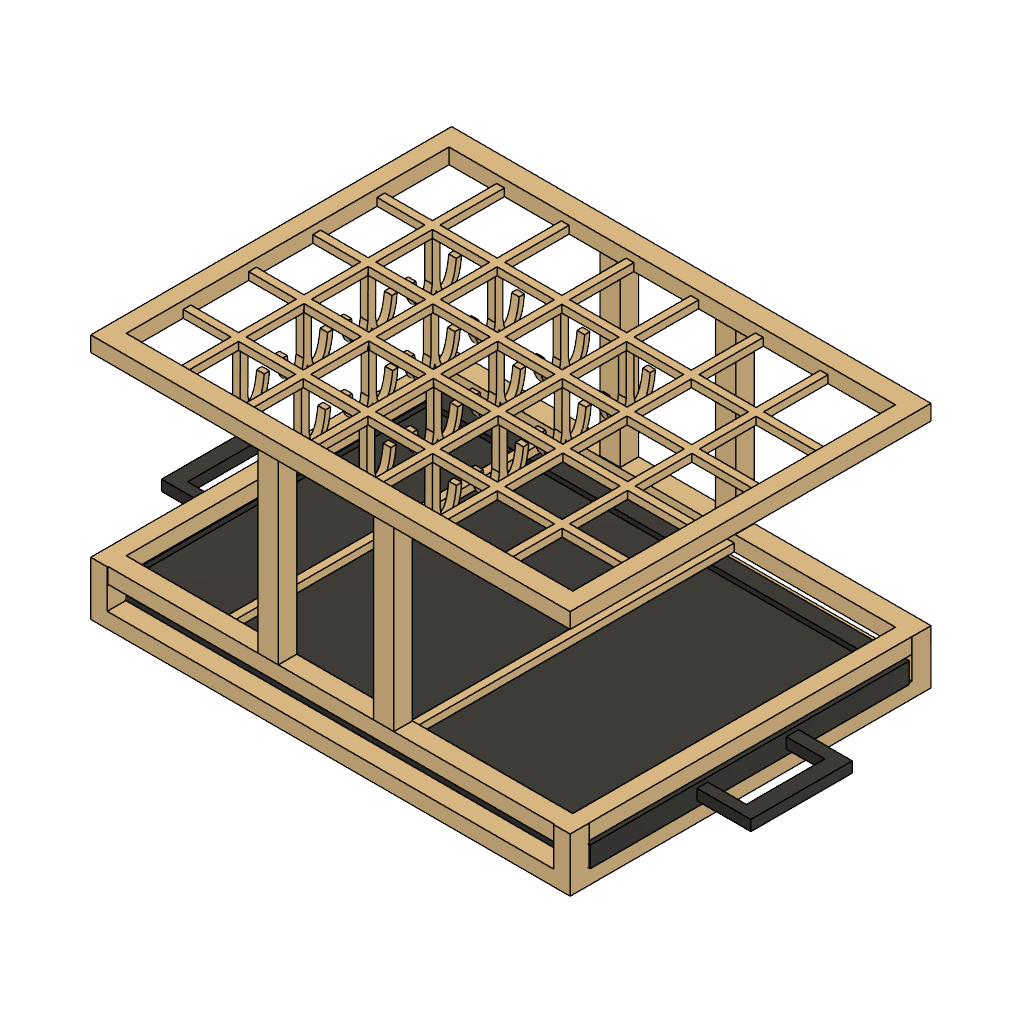
umbrella stand (Autodesk Fusion 360 design; units mm, degrees)
part number: 2026-07-15-13-42-07-009
Autodesk Fusion 360 part; units mm, degrees
note: some values were not read from the file. Chosen so that the rebuilt part matches the saved one: which bodies a step acts on; which face or edge a step refers to.
sketch "Sketch1" plane through (0, 0, 0) normal (0, 1, 0) x (1, 0, 0)
  line L0 (311.1189, -234.2212) -> (-311.1189, -234.2212)
  line L1 (-311.1189, -234.2212) -> (-311.1189, 234.2212)
  line L2 (-311.1189, 234.2212) -> (311.1189, 234.2212)
  line L3 (311.1189, 234.2212) -> (311.1189, -234.2212)
  line L4 (311.1189, -234.2212) -> (-311.1189, 234.2212) construction
  line L5 (-311.1189, -234.2212) -> (311.1189, 234.2212) construction
  line L6 (289.6996, -209.3887) -> (-289.6996, -209.3887)
  line L7 (-289.6996, -209.3887) -> (-289.6996, 209.3887)
  line L8 (-289.6996, 209.3887) -> (289.6996, 209.3887)
  line L9 (289.6996, 209.3887) -> (289.6996, -209.3887)
  line L10 (289.6996, -209.3887) -> (-289.6996, 209.3887) construction
  line L11 (-289.6996, -209.3887) -> (289.6996, 209.3887) construction
  line L12 (289.6996, -209.3887) -> (289.6996, -234.2212)
  line L13 (289.6996, -209.3887) -> (311.1189, -209.3887)
  line L14 (-289.6996, -209.3887) -> (-311.1189, -209.3887)
  line L15 (-311.1189, -209.3887) -> (-311.1189, -234.2212)
  line L16 (-311.1189, -234.2212) -> (-289.6996, -234.2212)
  line L17 (-289.6996, -234.2212) -> (-289.6996, -209.3887)
  line L18 (-289.6996, 209.3887) -> (-311.1189, 209.3887)
  line L19 (-311.1189, 209.3887) -> (-311.1189, 234.2212)
  line L20 (-311.1189, 234.2212) -> (-289.6996, 234.2212)
  line L21 (-289.6996, 234.2212) -> (-289.6996, 209.3887)
  line L22 (289.6996, 209.3887) -> (311.1189, 209.3887)
  line L23 (311.1189, 209.3887) -> (311.1189, 234.2212)
  line L24 (311.1189, 234.2212) -> (289.6996, 234.2212)
  line L25 (289.6996, 234.2212) -> (289.6996, 209.3887)
  constraint horizontal L0
  constraint perpendicular L0 L1
  constraint parallel L0 L2
  constraint parallel L1 L3
  constraint coincident L4 origin
  constraint coincident L5 origin
  constraint horizontal L6
  constraint perpendicular L6 L7
  constraint parallel L6 L8
  constraint parallel L7 L9
  constraint coincident L10 origin
  constraint coincident L11 origin
  constraint coincident L0 L12.end
  constraint perpendicular L0 L12
  constraint coincident L3 L13.end
  constraint perpendicular L3 L13
  constraint horizontal L14
  constraint vertical L15
  constraint horizontal L16
  constraint vertical L17
  constraint horizontal L18
  constraint vertical L19
  constraint horizontal L20
  constraint vertical L21
  constraint horizontal L22
  constraint vertical L23
  constraint horizontal L24
  constraint vertical L25
sketch "Sketch2" plane through (0, 0, 0) normal (0, 1, 0) x (1, 0, 0)
  line L0 (289.429, 6.0189) -> (-289.8763, 6.0189)
  line L1 (-289.8763, 6.0189) -> (-289.8763, 16.0189)
  line L2 (-289.8763, 16.0189) -> (289.429, 16.0189)
  line L3 (289.429, 16.0189) -> (289.429, 6.0189)
  line L4 (78, 210) -> (88, 210)
  line L5 (88, 210) -> (88, -209.6346)
  line L6 (88, -209.6346) -> (78, -209.6346)
  line L7 (78, -209.6346) -> (78, 210)
  line L8 (191.4008, 210) -> (201.4008, 210)
  line L9 (201.4008, 210) -> (201.4008, -209.2657)
  line L10 (201.4008, -209.2657) -> (191.4008, -209.2657)
  line L11 (191.4008, -209.2657) -> (191.4008, 210)
  line L12 (-289.8763, 126.0189) -> (289.429, 126.0189)
  line L13 (289.429, 126.0189) -> (289.429, 116.0189)
  line L14 (289.429, 116.0189) -> (-289.8763, 116.0189)
  line L15 (-289.8763, 116.0189) -> (-289.8763, 126.0189)
  line L16 (289.429, -118.9811) -> (-289.8763, -118.9811)
  line L17 (-289.8763, -118.9811) -> (-289.8763, -108.9811)
  line L18 (-289.8763, -108.9811) -> (289.429, -108.9811)
  line L19 (289.429, -108.9811) -> (289.429, -118.9811)
  line L20 (-42, 210) -> (-42, -209.6346)
  line L21 (-42, -209.6346) -> (-52, -209.6346)
  line L22 (-52, -209.6346) -> (-52, 210)
  line L23 (-52, 210) -> (-42, 210)
  line L24 (-157, 210) -> (-157, -209.6346)
  line L25 (-157, -209.6346) -> (-167, -209.6346)
  line L26 (-167, -209.6346) -> (-167, 210)
  line L27 (-167, 210) -> (-157, 210)
  line L28 (-280, 210) -> (-280, -209.6346)
  line L29 (-280, -209.6346) -> (-290, -209.6346)
  line L30 (-290, -209.6346) -> (-290, 210)
  line L31 (-290, 210) -> (-280, 210)
  line L32 (289.429, 116.0189, 300) -> (-289.8763, 116.0189, 300)
  line L33 (-289.8763, 116.0189, 300) -> (-289.8763, 126.0189, 300)
  line L34 (-289.8763, 126.0189, 300) -> (289.429, 126.0189, 300)
  line L35 (289.429, 126.0189, 300) -> (289.429, 116.0189, 300)
  dimension "d1" = 10
  dimension "d2" = 10
  dimension "d3" = 10
  dimension "d17" = 10
  dimension "d18" = 10
  dimension "d19" = 10
  dimension "d20" = 10
  dimension "d21" = 10
  dimension "d30" = 10
  constraint horizontal L0
  constraint vertical L1
  constraint horizontal L2
  constraint vertical L3
  constraint horizontal L4
  constraint vertical L5
  constraint horizontal L6
  constraint vertical L7
  constraint horizontal L8
  constraint vertical L9
  constraint horizontal L10
  constraint vertical L11
  constraint horizontal L14
  constraint vertical L15
  constraint horizontal L12
  constraint vertical L13
  constraint horizontal L16
  constraint vertical L17
  constraint horizontal L18
  constraint vertical L19
  constraint horizontal L23
  constraint vertical L20
  constraint horizontal L21
  constraint vertical L22
  constraint horizontal L27
  constraint vertical L24
  constraint horizontal L25
  constraint vertical L26
  constraint horizontal L31
  constraint vertical L28
  constraint horizontal L29
  constraint vertical L30
  measures "d1" distance of L0.start L2.end
  measures "d2" distance of L4.start L4.end
  measures "d3" distance of L8.start L8.end
  measures "d17" distance of L13.end L12.end
  measures "d18" distance of L16.start L18.end
  measures "d19" distance of L20.start L22.end
  measures "d20" distance of L24.start L26.end
  measures "d21" distance of L28.start L30.end
  measures "d30" distance of L12.end L13.end
ref_plane "WorkPlane1" through (0, 50, 0) normal (0, 1, 0) x (1, 0, 0)
sketch "Sketch3" plane through (0, 50, 0) normal (0, 1, 0) x (1, 0, 0)
  line L0 (-311.2382, 234.3503) -> (310.9801, 234.3503)
  line L1 (310.9801, 234.3503) -> (310.9801, -233.4061)
  line L2 (310.9801, -233.4061) -> (-311.2382, -233.4061)
  line L3 (-311.2382, -233.4061) -> (-311.2382, 234.3503)
  line L4 (-289.7, 209.4) -> (289.7, 209.4)
  line L5 (289.7, 209.4) -> (289.7, -209.39)
  line L6 (289.7, -209.39) -> (-289.7, -209.39)
  line L7 (-289.7, -209.39) -> (-289.7, 209.4)
  line L8 (310.9801, -233.4061) -> (289.7, -233.4061)
  line L9 (289.7, -233.4061) -> (289.7, -209.39)
  line L10 (289.7, -209.39) -> (310.9801, -209.39)
  line L11 (310.9801, -209.39) -> (310.9801, -233.4061)
  line L12 (-289.7, -209.39) -> (-311.2382, -209.39)
  line L13 (-311.2382, -209.39) -> (-311.2382, -233.4061)
  line L14 (-311.2382, -233.4061) -> (-289.7, -233.4061)
  line L15 (-289.7, -233.4061) -> (-289.7, -209.39)
  line L16 (-289.7, 209.4) -> (-311.2382, 209.4)
  line L17 (-311.2382, 209.4) -> (-311.2382, 234.3503)
  line L18 (-311.2382, 234.3503) -> (-289.7, 234.3503)
  line L19 (-289.7, 234.3503) -> (-289.7, 209.4)
  line L20 (289.7, 209.4) -> (310.9801, 209.4)
  line L21 (310.9801, 209.4) -> (310.9801, 234.3503)
  line L22 (310.9801, 234.3503) -> (289.7, 234.3503)
  line L23 (289.7, 234.3503) -> (289.7, 209.4)
  constraint horizontal L0
  constraint vertical L1
  constraint horizontal L2
  constraint vertical L3
  constraint horizontal L4
  constraint vertical L5
  constraint horizontal L6
  constraint vertical L7
  constraint horizontal L8
  constraint vertical L9
  constraint horizontal L10
  constraint vertical L11
  constraint horizontal L12
  constraint vertical L13
  constraint horizontal L14
  constraint vertical L15
  constraint horizontal L16
  constraint vertical L17
  constraint horizontal L18
  constraint vertical L19
  constraint horizontal L20
  constraint vertical L21
  constraint horizontal L22
  constraint vertical L23
sketch "Sketch4" plane through (0, 50, 0) normal (0, 1, 0) x (1, 0, 0)
  line L0 (-167, 210) -> (-157, 210)
  line L1 (-157, 210) -> (-157, -210)
  line L2 (-157, -210) -> (-167, -210)
  line L3 (-167, -210) -> (-167, 210)
  line L4 (-51.7031, 209.3781) -> (-41.7031, 209.3781)
  line L5 (-41.7031, 209.3781) -> (-41.7031, -209.2653)
  line L6 (-41.7031, -209.2653) -> (-51.7031, -209.2653)
  line L7 (-51.7031, -209.2653) -> (-51.7031, 209.3781)
  line L8 (-289.6742, 6.0201) -> (290.0056, 6.0201)
  line L9 (290.0056, 6.0201) -> (290.0056, 16.0201)
  line L10 (290.0056, 16.0201) -> (-289.6742, 16.0201)
  line L11 (-289.6742, 16.0201) -> (-289.6742, 6.0201)
  line L12 (78.2969, -209.2653) -> (78.2969, 209.3781)
  line L13 (78.2969, 209.3781) -> (88.2969, 209.3781)
  line L14 (88.2969, 209.3781) -> (88.2969, -209.2653)
  line L15 (88.2969, -209.2653) -> (78.2969, -209.2653)
  line L16 (191.2969, -209.2653) -> (191.2969, 209.3781)
  line L17 (191.2969, 209.3781) -> (201.2969, 209.3781)
  line L18 (201.2969, 209.3781) -> (201.2969, -209.2653)
  line L19 (201.2969, -209.2653) -> (191.2969, -209.2653)
  line L20 (290.0056, 126.0201) -> (-289.6742, 126.0201)
  line L21 (-289.6742, 126.0201) -> (-289.6742, 116.0201)
  line L22 (290.0056, 116.0201) -> (290.0056, 126.0201)
  line L23 (-289.6742, 116.0201) -> (290.0056, 116.0201)
  line L24 (-289.6742, -118.9799) -> (290.0056, -118.9799)
  line L25 (290.0056, -118.9799) -> (290.0056, -108.9799)
  line L26 (290.0056, -108.9799) -> (-289.6742, -108.9799)
  line L27 (-289.6742, -108.9799) -> (-289.6742, -118.9799)
  line L28 (-282, 210) -> (-282, -210)
  line L29 (-282, -210) -> (-292, -210)
  line L30 (-292, -210) -> (-292, 210)
  line L31 (-292, 210) -> (-282, 210)
  dimension "d5" = 10
  dimension "d6" = 10
  dimension "d22" = 10
  dimension "d23" = 10
  dimension "d24" = 10
  dimension "d25" = 10
  constraint horizontal L0
  constraint vertical L1
  constraint horizontal L2
  constraint vertical L3
  constraint horizontal L4
  constraint vertical L5
  constraint horizontal L6
  constraint vertical L7
  constraint horizontal L8
  constraint vertical L9
  constraint horizontal L10
  constraint vertical L11
  constraint horizontal L13
  constraint vertical L14
  constraint horizontal L15
  constraint vertical L12
  constraint horizontal L17
  constraint vertical L18
  constraint horizontal L19
  constraint vertical L16
  constraint horizontal L23
  constraint vertical L22
  constraint horizontal L20
  constraint vertical L21
  constraint horizontal L24
  constraint vertical L25
  constraint horizontal L26
  constraint vertical L27
  constraint horizontal L31
  constraint vertical L28
  constraint horizontal L29
  constraint vertical L30
  measures "d5" distance of L4.start L4.end
  measures "d6" distance of L8.start L10.end
  measures "d22" distance of L12.end L13.end
  measures "d23" distance of L17.end L16.end
  measures "d24" distance of L21.end L20.end
  measures "d25" distance of L24.start L26.end
extrude "Extrude1" add sketch "Sketch1" along normal blind 20 contours L0 L3 L12 L13 | L0 L6 L12 L17 | L3 L9 L13 L22 | L0 L1 L14 L15 L16 L17 | L2 L3 L22 L23 L24 L25 | L1 L7 L14 L18 | L2 L8 L21 L25 | L1 L2 L18 L19 L20 L21 makes body 1
extrude "Extrude2" add sketch "Sketch2" along normal blind 10 separate body contours L0 L2 L3 L9 | L0 L2 L9 L11 | L0 L2 L5 L11 | L0 L5 L7 L18 | L0 L2 L5 L7 | L0 L2 L7 L20 | L2 L5 L7 L14 | L5 L7 L16 L18 | L0 L2 L20 L22 | L5 L7 L12 L14 | L5 L6 L7 L16 | L0 L2 L22 L24 | L4 L5 L7 L12 | L0 L18 L24 L26 | L0 L2 L24 L26 | L0 L2 L26 L28 | L2 L14 L24 L26 | L16 L18 L24 L26 | L0 L1 L2 L28 | L12 L14 L24 L26 | L16 L24 L25 L26 | L12 L24 L26 L27 makes body 2
extrude "Extrude3" add sketch "Sketch3" along normal blind 20 separate body contours L0 L3 L16 L17 L18 L19 | L0 L4 L19 L23 | L3 L7 L12 L16 | L0 L1 L20 L21 L22 L23 | L2 L3 L12 L13 L14 L15 | L1 L5 L10 L20 | L2 L6 L9 L15 | L1 L2 L8 L9 L10 L11 makes body 3
extrude "Extrude4" add sketch "Sketch4" along normal blind 10 separate body contours L0 L1 L3 L20 | L1 L3 L20 L23 | L1 L3 L10 L23 | L1 L3 L8 L10 | L1 L3 L8 L26 | L12 L14 L20 L23 | L12 L13 L14 L20 | L1 L3 L24 L26 | L10 L12 L14 L23 | L1 L2 L3 L24 | L8 L10 L12 L14 | L8 L12 L14 L26 | L12 L14 L24 L26 | L12 L14 L15 L24 makes body 4 at (-157, 56.6667, -70) makes body 5 at (78.2969, 53.3333, 69.7175)
extrude "Extrude5" add sketch "Sketch1" along normal blind 70 separate body contours L0 L3 L12 L13 | L0 L1 L14 L15 L16 L17 | L2 L3 L22 L23 L24 L25 | L1 L2 L18 L19 L20 L21 makes body 6 at (-311.1189, 23.3333, 225.9437) makes body 7 at (311.1189, 23.3333, 217.6662) makes body 8 at (-289.6996, 46.6667, -225.9437) makes body 9 at (289.6996, 23.3333, -225.9437)
ref_plane "WorkPlane2" through (-0.129, 70, -0.4721) normal (0, 1, 0) x (0, 0, 1)
sketch "Sketch5" plane through (0, 70, 0) normal (0, 1, 0) x (1, 0, 0)
  line L0 (-94.8096, -209.39, -20) -> (-68.4638, -209.39, -20)
  line L1 (-68.4638, -209.39, -20) -> (-68.4638, -233.405, -20)
  line L2 (-68.4638, -233.405, -20) -> (-94.8096, -233.405, -20)
  line L3 (-94.8096, -233.405, -20) -> (-94.8096, -209.39, -20)
  line L4 (289.7, -209.39, -20) -> (-289.7, -209.39, -20)
  line L5 (55.1904, -233.405, -20) -> (55.1904, -209.39, -20)
  line L6 (55.1904, -209.39, -20) -> (81.5362, -209.39, -20)
  line L7 (81.5362, -233.405, -20) -> (55.1904, -233.405, -20)
  line L8 (81.5362, -209.39, -20) -> (81.5362, -233.405, -20)
ref_plane "WorkPlane3" through (0, 300, 0) normal (0, 1, 0) x (0, 0, 1)
sketch "Sketch5 (curves -20 mm off its plane)" plane through (0, 50, 0) normal (0, 1, 0) x (1, 0, 0)
  line L0 (-94.8096, -209.39) -> (-68.4638, -209.39)
  line L1 (-68.4638, -209.39) -> (-68.4638, -233.405)
  line L2 (-68.4638, -233.405) -> (-94.8096, -233.405)
  line L3 (-94.8096, -233.405) -> (-94.8096, -209.39)
  line L4 (289.7, -209.39) -> (-289.7, -209.39)
  line L5 (55.1904, -233.405) -> (55.1904, -209.39)
  line L6 (55.1904, -209.39) -> (81.5362, -209.39)
  line L7 (81.5362, -233.405) -> (55.1904, -233.405)
  line L8 (81.5362, -209.39) -> (81.5362, -233.405)
extrude "Extrude6" add sketch "Sketch5 (curves -20 mm off its plane)" along normal blind 250 separate body makes body 10 at (72.7543, 133.3333, 233.405) makes body 11 at (-86.0277, 133.3333, 209.39)
move_body "Move1" bodies 10 11 to x (1, 0, 0) y (0, 1, 0) z (0, 0, 1) at (0, 0, -443.75)
copy_body "CopyPasteBodies1" bodies 11 10 makes body 12 makes body 13
move_body "Move2" bodies 12 13 to x (1, 0, 0) y (0, 1, 0) z (0, 0, 1) at (0, 0, 443.75)
copy_body "CopyPasteBodies2" bodies 1 makes body 14
move_body "Move3" bodies 14 to x (1, 0, 0) y (0, 1, 0) z (0, 0, 1) at (0, 300, 0)
sketch "Sketch2 (curves 300 mm off its plane)" plane through (0, 300, 0) normal (0, 1, 0) x (1, 0, 0)
  line L0 (289.429, 116.0189) -> (-289.8763, 116.0189)
  line L1 (-289.8763, 116.0189) -> (-289.8763, 126.0189)
  line L2 (-289.8763, 126.0189) -> (289.429, 126.0189)
  line L3 (289.429, 126.0189) -> (289.429, 116.0189)
extrude "Extrude7" add sketch "Sketch2 (curves 300 mm off its plane)" along normal blind 10 separate body makes body 15
pattern_linear "R-Pattern1" count 4 spacing 83.3333 along (0, 0, 1) of bodies 15 makes body 16 at (96.3272, 303.3333, -32.6855) makes body 17 at (96.3272, 303.3333, 50.6478) makes body 18 at (96.3272, 303.3333, 133.9811)
move_body "Move4" bodies 18 to x (0, 0, 1) y (0, 1, 0) z (-1, 0, 0) at (326.1451, 0, -77.1829)
extrude "Extrude8" cut 1 faces at (195.4973, 303.3333, -367.0592) along direction (0, 0, 1) blind 135 on bodies 18 bodies 18
copy_body "CopyPasteBodies3" bodies 17 makes body 19
move_body "Move5" bodies 19 to x (1, 0, 0) y (0, 1, 0) z (0, 0, 1) at (0, 0, 75)
pattern_linear "R-Pattern2" count 6 spacing 84 along (-1, 0, 0) of bodies 18 makes body 20 at (114.8306, 300, -83.9574) makes body 21 at (30.8306, 300, -83.9574) makes body 22 at (-53.1694, 300, -83.9574) makes body 23 at (-137.1694, 300, -83.9574) makes body 24 at (-221.1694, 300, -83.9574)
move_body "Move6" bodies 19 to x (1, 0, 0) y (0, 1, 0) z (0, 0, 1) at (0, 0, 10)
ref_plane "WorkPlane4" through (311.1189, 10, 0) normal (1, 0, 0) x (0, 0, -1)
sketch "Sketch6" plane through (311.1189, 0, 0) normal (1, 0, 0) x (0, 0, -1)
  line L0 (-206.5339, 48.126) -> (207.4068, 48.126)
  line L1 (207.4068, 48.126) -> (207.4068, 21.4924)
  line L2 (207.4068, 21.4924) -> (-206.5339, 21.4924)
  line L3 (-206.5339, 21.4924) -> (-206.5339, 48.126)
  constraint horizontal L0
  constraint vertical L1
  constraint horizontal L2
  constraint vertical L3
extrude "Extrude9" add sketch "Sketch6" along normal blind 625 separate body makes body 25
move_body "Move7" bodies 25 to x (1, 0, 0) y (0, 1, 0) z (0, 0, 1) at (-600, 0, -500)
shell "Shell1" thickness 20 removed faces 1 at (-80.5478, 48.126, -431.4463) on bodies 25
ref_plane "WorkPlane5" through (336.1189, 34.8092, -500.4364) normal (1, 0, 0) x (0, 0, -1)
sketch "Sketch7" plane through (336.1189, 0, 0) normal (1, 0, 0) x (0, 0, -1)
  line L0 (431.9459, 42.5824) -> (563.7507, 42.5824)
  line L1 (563.7507, 42.5824) -> (563.7507, 28.7889)
  line L2 (563.7507, 28.7889) -> (431.9459, 28.7889)
  line L3 (431.9459, 28.7889) -> (431.9459, 42.5824)
  line L4 (431.9459, 42.5824) -> (445.9879, 42.5824)
  line L5 (445.9879, 42.5824) -> (445.9879, 28.7889)
  line L6 (445.9879, 28.7889) -> (431.9459, 28.7889)
  line L7 (431.9459, 28.7889) -> (431.9459, 42.5824)
  line L8 (563.7507, 42.5824) -> (547.9155, 42.5824)
  line L9 (547.9155, 42.5824) -> (547.9155, 28.7889)
  line L10 (547.9155, 28.7889) -> (563.7507, 28.7889)
  line L11 (563.7507, 28.7889) -> (563.7507, 42.5824)
  constraint horizontal L0
  constraint vertical L1
  constraint horizontal L2
  constraint vertical L3
  constraint horizontal L4
  constraint vertical L5
  constraint horizontal L6
  constraint vertical L7
  constraint coincident L2 L5.end
  constraint horizontal L8
  constraint vertical L9
  constraint horizontal L10
  constraint vertical L11
  constraint coincident L2 L9.end
combine "Combine1" operation add target body 14 tool bodies 11 7 5 15 12 2 4 19 6 1 16 3 22 13 17 8 24 9 20 21 23 10 18 makes body 26 at (78.2969, 53.3333, 69.7175)
move_body "Move8" bodies 26 to x (1, 0, 0) y (0, 1, 0) z (0, 0, 1) at (-7.8489, 0, -18.8738)
extrude "Extrude10" add 1 faces at (77.1146, 53.3333, 190.3915) along direction (0, 0, 1) blind 35 on bodies 26 bodies 14 26
extrude "Extrude11" add sketch "Sketch7" along normal blind 50 separate body contours L0 L2 L3 L4 L5 L6 L7 | L0 L1 L2 L8 L9 L10 L11 makes body 27 at (352.7856, 28.7889, -441.3072) makes body 28 at (352.7856, 42.5824, -553.1939)
extrude "Extrude12" add sketch "Sketch7" along normal blind 70 and the other way blind -50 bodies 25 14 27 28
copy_body "CopyPasteBodies4" bodies 27 makes body 30
move_body "Move9" bodies 30 to x (-1, 0, 0) y (0, -1, 0) z (0, 0, 1) at (52.2378, 71.3713, 0)
move_body "Move10" bodies 30 to x (1, 0, 0) y (0, 1, 0) z (0, 0, 1) at (-5, 0, 0)
combine "Combine3" operation add target body 27 tool bodies 30 25
sketch "Sketch8" plane through (0, 0, 0) normal (1, 0, 0) x (0, 0, -1)
  line L0 (-9.9869, -70) -> (0.0131, -70)
  line L1 (0.0131, -70) -> (0.0131, -95.6382)
  line L2 (0.0131, -95.6382) -> (-9.9869, -95.6382)
  line L3 (-9.9869, -95.6382) -> (-9.9869, -70)
  spline S0 degree 5 poles (-9.9869, -95.6382) (-10.0198, -95.9878) (-10.0891, -96.6913) (-10.204, -97.7592) (-10.3792, -99.2086) (-10.6409, -101.0592) (-10.9632, -102.936) (-11.3806, -104.8132) (-11.9514, -106.6463) (-12.7388, -108.3729) (-13.7915, -109.9132) (-15.1255, -111.1706) (-16.7016, -112.0312) (-18.4428, -112.3759) (-20.2574, -112.0942) (-22.0592, -111.0989) (-23.7867, -109.338) (-25.3965, -106.785) (-26.8605, -103.4323) (-28.1624, -99.2845) (-29.2943, -94.3529) (-30.0622, -89.7912) (-30.561, -86.028) (-30.8593, -83.3679) (-31, -82) knots 0 0 0 0 0 0 0.05 0.1 0.15 0.2 0.25 0.3 0.35 0.4 0.45 0.5 0.55 0.6 0.65 0.7 0.75 0.8 0.85 0.9 0.95 1 1 1 1 1 1
  spline S1 degree 5 poles (-4.9869, -95.6382) (-4.9116, -96.0837) (-4.7783, -96.9814) (-4.6301, -98.3472) (-4.5368, -100.2074) (-4.6005, -102.5923) (-4.8634, -105.0194) (-5.3599, -107.4533) (-6.1476, -109.8325) (-7.2915, -112.0762) (-8.8407, -114.0927) (-10.8109, -115.7883) (-13.1571, -117.0756) (-15.7729, -117.8807) (-18.522, -118.1466) (-21.2613, -117.8378) (-23.8667, -116.945) (-26.261, -115.4913) (-28.4075, -113.5245) (-30.2983, -111.1067) (-31.9443, -108.3056) (-33.3649, -105.1853) (-34.5773, -101.7963) (-35.595, -98.1758) (-36.4282, -94.3496) (-37.0841, -90.3344) (-37.4707, -86.9786) (-37.6841, -84.3827) (-37.7924, -82.6172) (-37.838, -81.7256) knots 0 0 0 0 0 0 0.04 0.08 0.12 0.16 0.2 0.24 0.28 0.32 0.36 0.4 0.44 0.48 0.52 0.56 0.6 0.64 0.68 0.72 0.76 0.8 0.84 0.88 0.92 0.96 1 1 1 1 1 1
  line L4 (-37.838, -81.7256) -> (-31, -82)
  spline S2 degree 5 poles (-5.0794, -95.6382) (-5.1548, -96.0837) (-5.2881, -96.9814) (-5.4362, -98.3472) (-5.5296, -100.2074) (-5.4659, -102.5923) (-5.203, -105.0194) (-4.7065, -107.4533) (-3.9188, -109.8325) (-2.7749, -112.0762) (-1.2257, -114.0927) (0.7445, -115.7883) (3.0907, -117.0756) (5.7065, -117.8807) (8.4556, -118.1466) (11.1949, -117.8378) (13.8004, -116.945) (16.1946, -115.4913) (18.3411, -113.5245) (20.2319, -111.1067) (21.8779, -108.3056) (23.2985, -105.1853) (24.5109, -101.7963) (25.5286, -98.1758) (26.3618, -94.3496) (27.0177, -90.3344) (27.4043, -86.9786) (27.6177, -84.3827) (27.726, -82.6172) (27.7717, -81.7256) knots 0 0 0 0 0 0 0.04 0.08 0.12 0.16 0.2 0.24 0.28 0.32 0.36 0.4 0.44 0.48 0.52 0.56 0.6 0.64 0.68 0.72 0.76 0.8 0.84 0.88 0.92 0.96 1 1 1 1 1 1
  spline S3 degree 5 poles (-0.0794, -95.6382) (-0.0466, -95.9878) (0.0227, -96.6913) (0.1376, -97.7592) (0.3128, -99.2086) (0.5745, -101.0592) (0.8968, -102.936) (1.3142, -104.8132) (1.885, -106.6463) (2.6724, -108.3729) (3.7251, -109.9132) (5.0592, -111.1706) (6.6352, -112.0312) (8.3764, -112.3759) (10.191, -112.0942) (11.9928, -111.0989) (13.7203, -109.338) (15.3301, -106.785) (16.7941, -103.4323) (18.096, -99.2845) (19.2279, -94.3529) (19.9958, -89.7912) (20.4946, -86.028) (20.793, -83.3679) (20.9336, -82) knots 0 0 0 0 0 0 0.05 0.1 0.15 0.2 0.25 0.3 0.35 0.4 0.45 0.5 0.55 0.6 0.65 0.7 0.75 0.8 0.85 0.9 0.95 1 1 1 1 1 1
  line L5 (27.7717, -81.7256) -> (20.9336, -82)
  point P0 (-11, -103)
  point P1 (-14, -110)
  point P2 (-20, -112)
  point P3 (-5, -105.4864)
  point P4 (-10, -115)
  point P5 (-21.6565, -117.5877)
  point P6 (-32.2294, -107.549)
  point P7 (-0.0664, -115)
  point P8 (11.5901, -117.5877)
  point P9 (0.9336, -103)
  point P10 (-5.0664, -105.4864)
  point P11 (22.163, -107.549)
  point P12 (9.9336, -112)
  point P13 (3.9336, -110)
  dimension "d56" = 10
  constraint horizontal L0
  constraint vertical L1
  constraint horizontal L2
  constraint vertical L3
  constraint midpoint L2 S1.start
  measures "d56" distance of L0.start L0.end
extrude "Extrude13" add sketch "Sketch8" along normal mid plane 10 separate body makes body 31
extrude "Extrude14" add 2 faces at (1.6667, -70, 6.6536) (-1.6667, -70, 6.6536) along direction (0, 1, 0) blind 30 on bodies 31 bodies 31
move_body "Move11" bodies 31 to x (1, 0, 0) y (0, 1, 0) z (0, 0, 1) at (-227.836, 370, 35.6608)
move_body "Move12" bodies 31 to x (0.996195, -0.087156, 0) y (0.087156, 0.996195, 0) z (0, 0, 1) at (-22.8365, -19.3346, 5)
move_body "Move13" bodies 31 to x (1, 0, 0) y (0, 1, 0) z (0, 0, 1) at (0.7813, -25.4905, 0.4555)
move_body "Move16" bodies 31 to x (0.996195, 0.086835, 0.007438) y (-0.08683, 0.996223, -0.000978) z (-0.007494, 0.000328, 0.999972) at (23.4201, 20.798, 1.9644)
copy_body "CopyPasteBodies5" bodies 31 makes body 32
move_body "Move17" bodies 32 to x (1, 0, 0) y (0, 1, 0) z (0, 0, 1) at (84.9976, -0.0273, 0.637)
copy_body "CopyPasteBodies6" bodies 32 makes body 33
move_body "Move18" bodies 33 to x (1, 0, 0) y (0, 1, 0) z (0, 0, 1) at (83.4299, -4.4849, -1.108)
copy_body "CopyPasteBodies7" bodies 33 makes body 34
move_body "Move19" bodies 34 to x (1, 0, 0) y (0, 1, 0) z (0, 0, 1) at (82.7, 0.2534, -2.4951)
pattern_linear "R-Pattern5" count 3 spacing 80 along (0, 0, -1) of bodies 34 makes body 35 at (33.3999, 261.5084, -38.4208) makes body 36 at (33.3999, 261.5084, -118.4208)
move_body "Move20" bodies 35 to x (1, 0, 0) y (0, 1, 0) z (0, 0, 1) at (-0.561, -1.7817, -1.7644)
move_body "Move21" bodies 36 to x (1, 0, 0) y (0, 1, 0) z (0, 0, 1) at (0.0341, 1.1511, -4.4993)
pattern_linear "R-Pattern6" count 3 spacing 85 along (-1, 0, 0) of bodies 35 makes body 37 at (-52.1611, 259.7267, -40.1851) makes body 38 at (-137.1611, 259.7267, -40.1851)
pattern_linear "R-Pattern7" count 3 spacing 85 along (-1, 0, 0) of bodies 36 makes body 39 at (-51.566, 262.6594, -122.9201) makes body 40 at (-136.566, 262.6594, -122.9201)
pattern_linear "R-Pattern8" count 2 spacing 87 along (0, 0, 1) of bodies 34 makes body 41
pattern_linear "R-Pattern9" count 3 spacing 85 along (-1, 0, 0) of bodies 41 makes body 42 at (-51.6001, 261.5084, 128.5792) makes body 43 at (-136.6001, 261.5084, 128.5792)
pattern_linear "R-Pattern10" count 3 spacing 83.5 along (0, 0, -1) of bodies 31 makes body 44 at (-217.7275, 265.7672, -38.9547) makes body 45 at (-217.7275, 265.7672, -122.4547)
copy_body "CopyPasteBodies8" bodies 43 makes body 46
move_body "Move22" bodies 46 to x (1, 0, 0) y (0, 1, 0) z (0, 0, 1) at (-79.9977, 0.0257, -0.5996)
combine "Combine4" operation add target body 39 tool bodies 43 14 34 44 35 32 31 41 42 46 40 33 36 37 38 45 makes body 47 at (32.8389, 259.7267, -40.1851) makes body 48 at (-137.1611, 259.7267, -40.1851) makes body 49 at (-49.3001, 261.255, 44.0744) makes body 50 at (-52.1611, 259.7267, -40.1851)
move_body "Move23" bodies 47 to x (1, 0, 0) y (0, 1, 0) z (0, 0, 1) at (0, 5, 0)
combine "Combine5" operation add target body 39 tool bodies 47 48 49 50 makes body 51 at (-49.3001, 261.255, 44.0744) makes body 52 at (-137.1611, 259.7267, -40.1851) makes body 53 at (-52.1611, 259.7267, -40.1851)
move_body "Move24" bodies 51 to x (1, 0, 0) y (0, 1, 0) z (0, 0, 1) at (0, 5, 0)
move_body "Move25" bodies 52 to x (1, 0, 0) y (0, 1, 0) z (0, 0, 1) at (0, 5, 0)
move_body "Move26" bodies 53 to x (1, 0, 0) y (0, 1, 0) z (0, 0, 1) at (0, 5, 0)
combine "Combine6" operation add target body 39 tool bodies 51 52 53
move_body "Move27" bodies 27 to x (1, 0, 0) y (0, 1, 0) z (0, 0, 1) at (-22.2378, -0.6857, 354.362)
move_body "Move28" bodies 27 to x (1, 0, 0) y (0, 1, 0) z (0, 0, 1) at (0, 0, 150)
scale "Scale1" factor 0.3 about (-291.1189, 40.8068, 190.8959) bodies 39 27
named bodies: "main", "tray", "Trey", "main"
